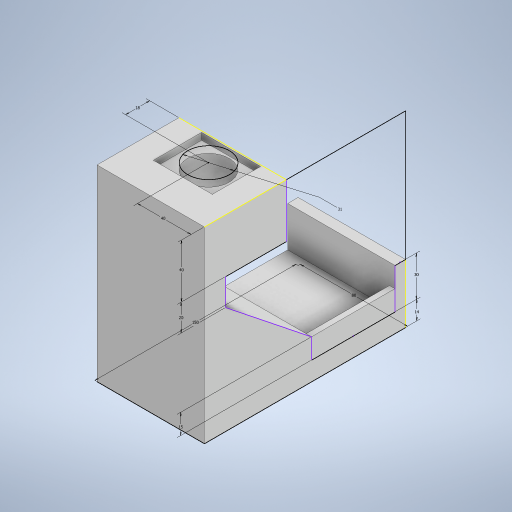
# Autodesk Inventor part: Left
Saved by Autodesk Inventor 2023.2 (Build 272271030, 271C)
## iProperties
Created: 2024-03-06
Part Number: Left
Material: Generic
Document SubType Name: Modeling
Designer: ryanv
Density: 1 g/cm^3
Appearance: Default
Author: ryanv
Autodesk Inventor part; units mm, degrees
ref_plane "YZ Plane" through (0, 0, 0) normal (1, 0, 0) x (0, 1, 0)
ref_plane "XZ Plane" through (0, 0, 0) normal (0, 1, 0) x (-1, 0, 0)
ref_plane "XY Plane" through (0, 0, 0) normal (0, 0, 1) x (1, 0, 0)
sketch "Sketch1" plane through (0, 0, 0) normal (0, 1, 0) x (-1, 0, 0)
  line L0 (0, 0) -> (80, 0)
  line L1 (80, 0) -> (80, -150)
  line L2 (80, -150) -> (0, -150)
  line L3 (0, -150) -> (0, 0)
  dimension "d0" = 80
  dimension "d1" = 150
  constraints: 8 end point, 2 parallel, 1 horizontal, 1 perpendicular
  measures "d0" distance of L1.end L2.end
  measures "d1" distance of L0.end L1.end
extrude "Extrusion1" add sketch "Sketch1" along normal blind 140
sketch "Sketch2" plane through (0, 0, 0) normal (1, 0, 0) x (0, 0, -1)
  line L0 (150, 140) -> (0, 140) projected
  line L1 (61.0962, 140) -> (61.0962, 100)
  line L2 (61.0962, 100) -> (15.8986, 100)
  line L3 (15.8986, 80) -> (79.9832, 29)
  line L4 (79.9832, 29) -> (79.9832, 14)
  line L5 (79.9832, 14) -> (142.2187, 14)
  line L6 (142.2187, 14) -> (142.2187, 44)
  line L7 (142.2187, 44) -> (150, 44)
  line L8 (150, 0) -> (150, 140) projected
  line L9 (150, 44) -> (150, 140)
  line L10 (150, 140) -> (61.0962, 140)
  line L11 (15.8986, 100) -> (15.8986, 80)
  line L12 (0, 0) -> (150, 0) projected
  point P0 (146.1093, 44)
  point P1 (111.101, 14)
  dimension "d7" = 15
  dimension "d8" = 30
  dimension "d9" = 14
  dimension "d11" = 40
  dimension "d12" = 20
  constraints: 20 end point, 8 perpendicular, 2 midpoint, 1 point on line, 1 vertical
  measures "d7" distance from line of L5 L3.end
  measures "d8" distance from line of L5 point (146.109, 44)
  measures "d9" distance from line of L12 point (111.101, 14)
  measures "d11" distance between parallel lines of L0 L2
  measures "d12" distance from line of L3.start L2
extrude "Extrusion2" cut sketch "Sketch2" against normal blind 140
sketch "Sketch3" plane through (0, 14, -79.9832) normal (0, 1, 0) x (1, 0, 0)
  line L0 (0, -79.9832) -> (0, 70.0168) projected
  line L1 (0, 0) -> (-80, 0) projected
  line L2 (0, 62.5105) -> (-4, 62.5105)
  line L3 (-4, 62.5105) -> (-4, 0)
  line L4 (-4, 0) -> (0, 0)
  line L5 (0, 0) -> (0, 62.5105)
  dimension "d13" = 4
  constraints: 8 end point, 2 parallel, 2 point on line, 1 horizontal, 1 perpendicular
  measures "d13" distance between parallel lines of L3 L0
extrude "Extrusion3" add sketch "Sketch3" along normal blind 15
sketch "Sketch4" plane through (0, 140, 0) normal (0, 1, 0) x (1, 0, 0)
  circle A0 centre (-40, 43.0962) radius 15.5
  line L0 (0, 61.0962) -> (-80, 61.0962) projected
  line L1 (0, 0) -> (0, 61.0962) projected
  dimension "d18" = 31
  dimension "d19" = 18
  dimension "d20" = 40
  constraints: 1 centre point
  measures "d18" diameter of A0
  measures "d19" distance from line of A0.centre L0
  measures "d20" distance from line of L1 A0.centre
extrude "Extrusion4" cut sketch "Sketch4" against normal blind 50
sketch "Sketch5" plane through (0, 140, 0) normal (0, 1, 0) x (1, 0, 0)
  line L0 (-18, 24) -> (-62, 24)
  line L1 (-62, 24) -> (-62, 60)
  line L2 (-62, 60) -> (-18, 60)
  line L3 (-18, 60) -> (-18, 24)
  line L4 (-80, 61.0962) -> (-80, 0) projected
  line L5 (0, 0) -> (0, 61.0962) projected
  line L6 (-80, 0) -> (0, 0) projected
  line L7 (0, 61.0962) -> (-80, 61.0962) projected
  dimension "d21" = 36
  dimension "d22" = 18
  dimension "d23" = 18
  dimension "d26" = 24
  constraints: 8 end point, 2 parallel, 1 horizontal, 1 perpendicular
  measures "d21" distance between parallel lines of L2 L0
  measures "d22" distance between parallel lines of L4 L1
  measures "d23" distance between parallel lines of L5 L3
  measures "d26" distance between parallel lines of L6 L0
extrude "Extrusion5" cut sketch "Sketch5" against normal blind 5 contours L0 L1 L2 L3
body "Solid1"
